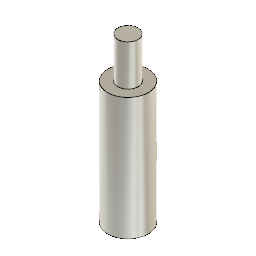
actuator v4 (Autodesk Fusion 360 design; units mm, degrees)
Autodesk Fusion 360 part; units mm, degrees
cylinder "CylinderPrimitive1" add diameter 20 height 60 placed x (1, 0, 0) y (0, 1, 0) z (0, 0, 1) at (0, 0, 0)
sketch "cut out" plane through (0, 0, 60) normal (0, 0, 1) x (-1, 0, 0)
  circle A0 centre (0, 0) radius 10
  circle A1 centre (0, 0) radius 5
  dimension "d3" = 10
  constraint coincident A0.centre A1.centre
  measures "d3" diameter of A1
extrude "Extrude1" cut sketch "cut out" against normal blind 40 contours A1
sketch "cylinder" plane through (0, 0, 20) normal (0, 0, 1) x (-1, 0, 0)
  circle A0 centre (0, 0) radius 5
  circle A1 centre (0, 0) radius 5
  constraint coincident A0.centre A1.centre
extrude "Extrude2" add sketch "cylinder" along normal blind 60
named bodies: "actuator body"
